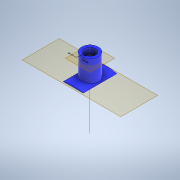
# Autodesk Inventor part: tubeBracketV03
Saved by Autodesk Inventor 2021 (Build 250183000, 183)
## iProperties
Created: 2020-05-27
Part Number: tubeBracketV03
Material: PC/ABS Plastic
Document SubType Name: Modeling
Designer: robst
Density: 0.357273 g/cm^3
Appearance: Blue - Wall Paint - Glossy
Author: robst
Autodesk Inventor part; units mm, degrees
ref_plane "YZ Plane" through (0, 0, 0) normal (1, 0, 0) x (0, 1, 0)
ref_plane "XY Plane" through (0, 0, 0) normal (0, 0, 1) x (1, 0, 0)
sketch "Sketch8" plane through (0, 0, 0) normal (0, 0, 1) x (1, 0, 0)
  arc A0 (76.1338, 3.175) -> (-76.1338, 3.175) centre (0, 0) ccw
  arc A1 (81.9986, 9.525) -> (-81.9986, 9.525) centre (0, 0) ccw
  line L0 (-82.4889, 3.175) -> (-101.5389, 3.175)
  line L1 (-101.5389, 3.175) -> (-101.5389, 9.525)
  line L2 (-101.5389, 9.525) -> (-81.9986, 9.525)
  line L3 (0, 0) -> (0, 82.55) construction
  line L4 (-82.4889, 3.175) -> (-76.1338, 3.175)
  line L5 (82.4889, 3.175) -> (101.5389, 3.175)
  line L6 (101.5389, 3.175) -> (101.5389, 9.525)
  line L7 (101.5389, 9.525) -> (81.9986, 9.525)
  line L8 (82.4889, 3.175) -> (76.1338, 3.175)
  dimension "d52" = 152.4
  dimension "d53" = 6.35
  dimension "d54" = 19.05
  dimension "d55" = 3.175
  dimension "d56" = 6.35
  constraints: 18 end point, 5 point on circle, 5 symmetric about line, 2 centre point, 2 coincident, 2 horizontal, 2 vertical, 1 perpendicular
  measures "d52" diameter of A0
  measures "d53" radial gap between concentric circles of A1 A0
  measures "d54" distance of L0.end L0.start
  measures "d55" distance from line of point (0, 0) L0
  measures "d56" distance of L0.end L1.end
extrude "Extrusion5" add sketch "Sketch8" along normal mid plane 76.2
sketch "Sketch9" plane through (-101.5389, 9.525, 38.1) normal (0, 1, 0) x (1, 0, 0)
  line L0 (19.5403, 0) -> (0, 0) construction
  line L1 (9.7701, 0) -> (9.7701, 76.2) construction
  line L2 (25.4051, 76.2) -> (0, 76.2) construction
  line L3 (9.7701, 25.4) -> (9.7701, 101.6) construction
  line L4 (9.7701, 50.8) -> (9.7701, 127) construction
  point P0 (101.5389, 38.1)
  point P1 (9.7701, 12.7)
  point P2 (9.7701, 38.1)
  point P3 (9.7701, 63.5)
  dimension "d59" = 12.7
  dimension "d62" = 25.4
  constraints: 6 end point, 4 point on line, 2 vertical, 1 collinear, 1 midpoint, 7 other
  measures "d59" distance of point (9.77, 12.7) L1.start
  measures "d62" distance of point (9.77, 12.7) point (9.77, 38.1)
hole "Hole3" at (-91.7688, 9.525, 25.4) at (-91.7688, 9.525, 0) at (-91.7688, 9.525, -25.4) direction (0, -1, 0) diameter 6.7564 end through all clearance for "Socket Head Cap Screw" size "1/4" standard "Ansi Unified Screw Threads"
mirror "Mirror3" about plane through (0, 0, 0) normal (1, 0, 0) of "Hole3"
ref_plane "Work Plane7" through (0, 79.375, 0) normal (0, 1, 0) x (-1, 0, 0)
sketch "Sketch20" plane through (0, 79.375, 0) normal (0, 1, 0) x (-1, 0, 0)
  circle A0 centre (0, 0) radius 19.05
  dimension "d101" = 38.1
  constraints: 1 centre point, 1 coincident
  measures "d101" diameter of A0
extrude "Extrusion11" add sketch "Sketch20" along normal blind 50.8
sketch "Sketch22" plane through (0, 130.175, 0) normal (0, 1, 0) x (1, 0, 0)
  circle A0 centre (0, 0) radius 12.7
  dimension "d111" = 25.4
  constraints: 1 centre point, 1 coincident
  measures "d111" diameter of A0
extrude "Extrusion13" cut sketch "Sketch22" against normal blind 50.8
sketch "Sketch23" plane through (0, 130.175, 0) normal (0, 1, 0) x (1, 0, 0)
  circle A0 centre (0, 0) radius 12.7 projected
  arc A1 (-1.5875, -12.6004) -> (1.5875, -12.6004) centre (0, 0) ccw
  arc A2 (-1.5875, -14.199) -> (1.5875, -14.199) centre (0, 0) ccw
  line L0 (0, 0) -> (0, -14.2875) construction
  line L1 (-1.5875, -12.6004) -> (-1.5875, -14.199)
  line L2 (1.5875, -12.6004) -> (1.5875, -14.199)
  point P0 (1.5875, -12.6004)
  dimension "d114" = 28.575
  dimension "d115" = 1.5875
  dimension "d116" = 1.5875
  dimension "d117" = 25.4
  constraints: 6 end point, 5 point on circle, 2 centre point, 2 coincident, 2 vertical, 1 parallel
  measures "d114" diameter of A2
  measures "d115" distance between parallel lines of L2 L0
  measures "d116" distance between parallel lines of L1 L0
  measures "d117" diameter of A1
extrude "Extrusion14" cut sketch "Sketch23" against normal blind 12.7 contours A0 L2 A2 L1
ref_plane "Work Plane9" through (0, 117.475, 0) normal (0, 1, 0) x (1, 0, 0)
sketch "Sketch24" plane through (0, 117.475, 0) normal (0, 1, 0) x (1, 0, 0)
  circle A0 centre (0, 0) radius 14.2875
  dimension "d121" = 28.575
  constraints: 1 centre point, 1 coincident
  measures "d121" diameter of A0
extrude "Extrusion15" cut sketch "Sketch24" against normal blind 12.7
sketch "Sketch25" plane through (0, 79.375, 0) normal (0, 1, 0) x (-1, 0, 0)
  line L0 (101.5389, -38.1) -> (101.5389, 38.1) projected
  line L1 (81.9986, 38.1) -> (101.5389, 38.1) projected
  line L2 (101.5389, -38.1) -> (81.9986, -38.1) projected
  line L3 (-81.9986, -38.1) -> (-101.5389, -38.1) projected
  line L4 (-101.5389, 38.1) -> (-81.9986, 38.1) projected
  line L5 (-101.5389, -38.1) -> (-101.5389, 38.1) projected
  line L6 (101.5389, -38.1) -> (101.5389, 38.1) projected
  line L7 (-101.5389, -38.1) -> (-76.1338, -38.1) projected
  line L8 (101.5389, 38.1) -> (-101.5389, 38.1)
  line L9 (-101.5389, 38.1) -> (-101.5389, -38.1)
  line L10 (-101.5389, -38.1) -> (101.5389, -38.1)
  line L11 (101.5389, -38.1) -> (101.5389, 38.1)
  point P0 (0, 0)
  constraints: 8 end point, 2 parallel, 1 horizontal, 1 perpendicular
extrude "Extrusion16" cut sketch "Sketch25" against normal blind 76.2
body "Solid3"
